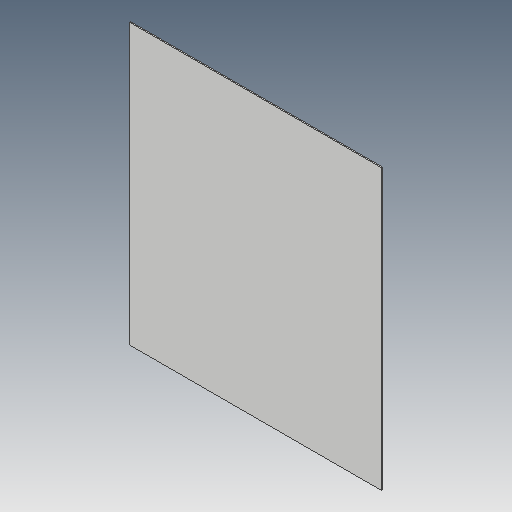
# Autodesk Inventor part: StandPlatform
Saved by Autodesk Inventor 2017 (Build 210142000, 142)
## iProperties
Created: 2017-05-22
Part Number: StandPlatform
Material: Generic
Document SubType Name: Modeling
Designer: krosie
Density: 1 g/cm^3
Appearance: Default
Author: krosie
Autodesk Inventor part; units mm, degrees
ref_plane "YZ Plane" through (0, 0, 0) normal (1, 0, 0) x (0, 1, 0)
ref_plane "XZ Plane" through (0, 0, 0) normal (0, 1, 0) x (-1, 0, 0)
ref_plane "XY Plane" through (0, 0, 0) normal (0, 0, 1) x (1, 0, 0)
sketch "Sketch1" plane through (0, 0, 0) normal (0, 0, 1) x (1, 0, 0)
  line L0 (-450, 0) -> (-450, 110) projected
  line L1 (0, 110) -> (0, 0) projected
  line L2 (0, -280) -> (0, -390) projected
  line L3 (-450, -390) -> (-450, -280) projected
  line L4 (-450, -390) -> (0, -390)
  line L5 (0, -390) -> (0, 110)
  line L6 (0, 110) -> (-450, 110)
  line L7 (-450, 110) -> (-450, -390)
  constraints: 8 end point, 2 parallel, 1 horizontal, 1 perpendicular
extrude "Extrusion1" add sketch "Sketch1" along normal blind 2
body "Solid1"
